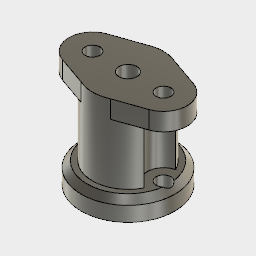
Titan Extruder Groove Mount Mosquito 3mm v3 (Autodesk Fusion 360 design; units mm, degrees)
Autodesk Fusion 360 part; units mm, degrees
sketch "Sketch1" plane through (0, 0, 0) normal (0, 0, 1) x (1, 0, 0)
  line L0 (0, 0) -> (25, 0)
  line L1 (25, 0) -> (25, -13)
  line L2 (25, -13) -> (0, -13)
  line L3 (0, -13) -> (0, 0)
  circle A0 centre (12.5, -6.5) radius 0.9
  circle A1 centre (6.5, -6.5) radius 1.25
  circle A2 centre (18.5, -6.5) radius 1.25
  line L4 (12.5, -6.5) -> (17, -6.5) construction
  circle A3 centre (18.5, -6.5) radius 2.75
  circle A4 centre (6.5, -6.5) radius 2.75
  circle A5 centre (18.5, -6.5) radius 4
  circle A6 centre (6.5, -6.5) radius 4
  circle A7 centre (12.5, -6.5) radius 6
  line L5 (15.0075, -11.9509) -> (19.8148, -10.2777)
  line L6 (9.9925, -11.9509) -> (5.1852, -10.2777)
  line L7 (9.9925, -1.0491) -> (5.1852, -2.7223)
  line L8 (15.0075, -1.0491) -> (19.8148, -2.7223)
  dimension "d1" = 25
  dimension "d2" = 13
  dimension "d3" = 1.8
  dimension "d7" = 2.5
  dimension "d8" = 2.5
  dimension "d12" = 5.5
  dimension "d13" = 5.5
  dimension "d14" = 8
  dimension "d15" = 8
  dimension "d16" = 12
  measures "d1" distance of L0.start L0.end
  measures "d2" distance of L0.start L2.end
  measures "d3" diameter of A0
  measures "d7" diameter of A1
  measures "d8" diameter of A2
  measures "d12" diameter of A3
  measures "d13" diameter of A4
  measures "d14" diameter of A5
  measures "d15" diameter of A6
  measures "d16" diameter of A7
extrude "Extrude1" add sketch "Sketch1" along normal blind 3 contours A1 A4 A7 | A1 A4 A7 | A4 A6 A7 | A4 A6 A7 | A5 A6 A7 | A6 A7 L7 | A6 A7 L6 | A5 A7 L8 | A5 A7 L5 | A3 A5 A7 | A3 A5 A7 | A2 A3 A7 | A2 A3 A7
extrude "Extrude2" cut sketch "Sketch1" along normal blind 0.5 contours A1 A4 A7 | A1 A4 A7
extrude "Extrude3" cut sketch "Sketch1" along normal blind 1 contours A1 A4 A7 | A1 A4 A7 | A2 A3 A7 | A2 A3 A7
extrude "Extrude4" add sketch "Sketch1" against normal blind 6 contours A4 A6 A7 | A5 A6 A7 | A3 A5 A7 picked at (7.9318, -3.3826) picked at (17.0587, -9.6124)
sketch "Sketch2" plane through (0, 0, -6) normal (0, 0, -1) x (1, 0, 0)
  circle A0 centre (12.5, 6.5) radius 0.9
  arc A1 (7.1302, 3.8232) -> (17.8698, 3.8232) centre (12.5, 6.5) ccw
  arc A2 (17.8698, 9.1768) -> (17.8698, 3.8232) centre (18.5, 6.5) ccw
  arc A3 (17.8698, 9.1768) -> (7.1302, 9.1768) centre (12.5, 6.5) ccw
  arc A4 (7.1302, 3.8232) -> (7.1302, 9.1768) centre (6.5, 6.5) ccw
  circle A5 centre (12.5, 6.5) radius 8
  dimension "d25" = 16
  measures "d25" diameter of A5
extrude "Extrude5" add sketch "Sketch2" along normal blind 3.5 contours A1 A2 A3 A4 | A5
extrude "Extrude6" cut sketch "Sketch1" against normal blind 12.5 contours A1 A7 | A1 A7 | A2 A7 | A2 A7
sketch "Sketch3" plane through (0, 0, -9.5) normal (0, 0, -1) x (1, 0, 0)
  circle A0 centre (18.5, 6.5) radius 1.25
  circle A1 centre (6.5, 6.5) radius 1.25
  circle A2 centre (12.5, 6.5) radius 0.9
  circle A3 centre (12.5, 6.5) radius 8
  circle A4 centre (12.5, 6.5) radius 2.1
  dimension "d30" = 4.2
  measures "d30" diameter of A4
extrude "Extrude7" cut sketch "Sketch3" against normal blind 19.5 contours A4
sketch "Sketch4" plane through (0, 0, -9.5) normal (0, 0, -1) x (1, 0, 0)
  circle A0 centre (12.5, 6.5) radius 2.1
  circle A1 centre (18.5, 6.5) radius 1.25
  circle A2 centre (6.5, 6.5) radius 1.25
  circle A3 centre (12.5, 6.5) radius 8
  circle A4 centre (12.5, 6.5) radius 7.9
  dimension "d33" = 15.8
  measures "d33" diameter of A4
extrude "Extrude8" cut sketch "Sketch4" against normal blind 4 contours A3
chamfer "Chamfer1" distance 1 angle 45 1 edges at (5.1346, -9.3568, -6)
extrude "Extrude9" add 1 faces at (9.4108, -3.8811, 3) along direction (0, 0, 1) blind 4
extrude "Extrude10" cut 2 faces at (8.7398, -6.3634, 1) (20.7351, -6.3013, 1) along direction (0, 0, 1) blind 4
extrude "Extrude11" cut 2 faces at (18.6335, -9.8007, 0) (6.3563, -3.1998, 0) along direction (0, 0, 1) blind 4
sketch "Sketch5" plane through (0, 0, 7) normal (0, 0, 1) x (-1, 0, 0)
  circle A0 centre (-12.5, 6.5) radius 2.1
  circle A1 centre (-18.5, 6.5) radius 1.25
  circle A2 centre (-6.5, 6.5) radius 1.25
  line L0 (-9.9925, 1.0491) -> (-5.1852, 2.7223)
  arc A3 (-5.1852, 2.7223) -> (-5.1852, 10.2777) centre (-6.5, 6.5) ccw
  line L1 (-5.1852, 10.2777) -> (-9.9925, 11.9509)
  arc A4 (-9.9925, 11.9509) -> (-15.0075, 11.9509) centre (-12.5, 6.5) ccw
  line L2 (-15.0075, 11.9509) -> (-19.8148, 10.2777)
  arc A5 (-19.8148, 10.2777) -> (-19.8148, 2.7223) centre (-18.5, 6.5) ccw
  line L3 (-19.8148, 2.7223) -> (-15.0075, 1.0491)
  arc A6 (-15.0075, 1.0491) -> (-9.9925, 1.0491) centre (-12.5, 6.5) ccw
  circle A7 centre (-12.5, 6.5) radius 1.5
  dimension "d43" = 3
  measures "d43" diameter of A7
extrude "Extrude12" add sketch "Sketch5" against normal blind 16.5 contours A0
